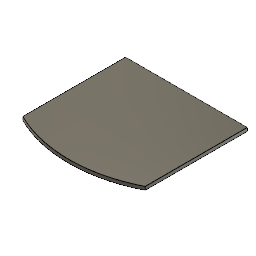
CurvyShelf v3 (Autodesk Fusion 360 design; units mm, degrees)
Autodesk Fusion 360 part; units mm, degrees
sketch "Sketch1" plane through (0, 0, 0) normal (0, 1, 0) x (1, 0, 0)
  line L0 (436.1445, 2.1916) -> (436.1445, 368.3)
  line L1 (436.1445, 368.3) -> (0, 368.3)
  line L2 (0, 368.3) -> (0, 0)
  arc A0 (0, 0) -> (436.1445, 2.1916) centre (215.9, 433.3875) ccw
  dimension "d1" = 368.3
  dimension "d2" = 436.15
  measures "d1" distance of L2.end L1.end
  measures "d2" distance of L2.end L0.start
extrude "Extrude2" add sketch "Sketch1" along normal blind 12.7
extrude "Extrude1" [suppressed]
